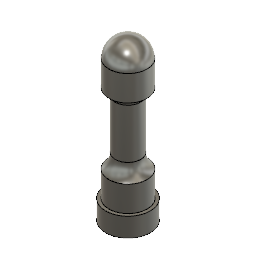
Task1c v0 (Autodesk Fusion 360 design; units mm, degrees)
Autodesk Fusion 360 part; units mm, degrees
sketch "Sketch1" plane through (0, 0, 0) normal (0, 1, 0) x (1, 0, 0)
  circle A0 centre (0, 0) radius 3.5
  dimension "d1" = 7
  constraint coincident A0.centre origin
  measures "d1" diameter of A0
extrude "Extrude1" add sketch "Sketch1" along normal blind 3
sphere "SpherePrimitive1" cut diameter 3 placed x (1, 0, 0) y (0, 0, -1) z (0, 1, 0) at (0, 0, 0)
sketch "Sketch4" plane through (0, 3, 0) normal (0, 1, 0) x (-1, 0, 0)
  circle A0 centre (0, 0) radius 3.5
  circle A1 centre (0, 0) radius 3
  dimension "d6" = 6
  constraint concentric A0 A1
  measures "d6" diameter of A1
extrude "Extrude2" add sketch "Sketch4" along normal blind 4 contours A1
sketch "Sketch5" plane through (0, 7, 0) normal (0, 1, 0) x (-1, 0, 0)
  circle A0 centre (0, 0) radius 3
  circle A1 centre (0, 0) radius 2
  dimension "d9" = 4
  constraint coincident A0.centre A1.centre
  measures "d9" diameter of A1
extrude "Extrude3" add sketch "Sketch5" along normal blind 11 contours A1
sketch "Sketch6" plane through (0, 18, 0) normal (0, 1, 0) x (-1, 0, 0)
  circle A0 centre (0, 0) radius 2
  circle A1 centre (0, 0) radius 3
  dimension "d12" = 6
  constraint concentric A0 A1
  measures "d12" diameter of A1
extrude "Extrude4" add sketch "Sketch6" along normal blind 7 contours A0 | A1
extrude "Extrude5" cut 1 faces at (1.1591, 25, 0.5829) along direction (0, -1, 0) blind 3
sphere "SpherePrimitive2" add diameter 6 placed x (-1, 0, 0) y (0, 0, 1) z (0, 1, 0) at (0, 22, 0)
fillet "Fillet1" radius 1 1 edges at (1.8647, 18, -0.7232)
fillet "Fillet2" radius 3 1 edges at (1.8647, 7, 0.7232)
sketch "Sketch2" plane through (0, 0, 0) normal (0, -1, 0) x (1, 0, 0)
  circle A0 centre (0, 0) radius 3.5
  circle A1 centre (0, 0) radius 1.5
  dimension "d4" = 3
  constraint concentric A0 A1
  measures "d4" diameter of A1
